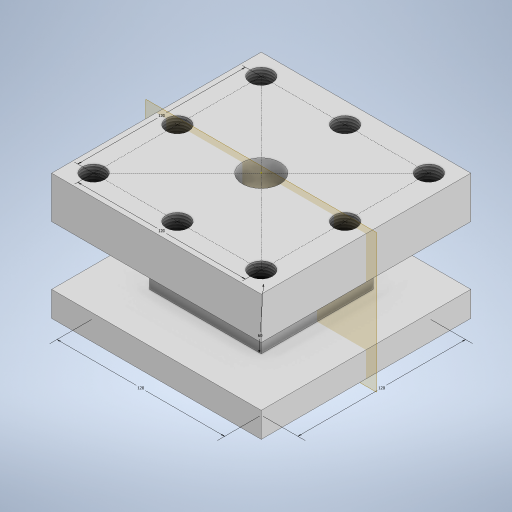
# Autodesk Inventor part: Body
Saved by Autodesk Inventor 2024 (Build 280153000, 153)
## iProperties
Created: 2023-11-09
Part Number: Body
Material: Generic
Document SubType Name: Modeling
Designer: Admin
Density: 1 g/cm^3
Appearance: Default
Author: Admin
Autodesk Inventor part; units mm, degrees
ref_plane "YZ Plane" through (0, 0, 0) normal (1, 0, 0) x (0, 1, 0)
ref_plane "XZ Plane" through (0, 0, 0) normal (0, 1, 0) x (-1, 0, 0)
sketch "Sketch1" plane through (0, 0, 0) normal (0, 1, 0) x (-1, 0, 0)
  line L0 (-75, -75) -> (75, -75)
  line L1 (75, -75) -> (75, 75)
  line L2 (75, 75) -> (-75, 75)
  line L3 (-75, 75) -> (-75, -75)
  line L4 (-75, -75) -> (75, 75) construction
  line L5 (75, -75) -> (-75, 75) construction
  point P0 (0, 0)
  dimension "d0" = 150
  dimension "d1" = 150
  constraints: 12 end point, 2 midpoint, 2 parallel, 1 horizontal, 1 perpendicular
  measures "d0" distance of L2.end L1.end
  measures "d1" distance of L1.end L0.end
extrude "Extrusion1" add sketch "Sketch1" against normal blind 18
sketch "Sketch2" plane through (0, -18, 0) normal (0, -1, 0) x (1, 0, 0)
  circle A0 centre (0, 0) radius 30
  line L0 (-60, -60) -> (60, -60) construction
  line L1 (60, -60) -> (60, 60) construction
  line L2 (60, 60) -> (-60, 60) construction
  line L3 (-60, 60) -> (-60, -60) construction
  line L4 (-60, -60) -> (60, 60) construction
  line L5 (60, -60) -> (-60, 60) construction
  dimension "d4" = 60
  dimension "d5" = 120
  dimension "d6" = 120
  constraints: 12 end point, 2 midpoint, 2 parallel, 1 centre point, 1 coincident, 1 horizontal, 1 perpendicular
  measures "d4" diameter of A0
  measures "d5" distance of L2.end L1.end
  measures "d6" distance of L1.end L0.end
extrude "Extrusion2" cut sketch "Sketch2" against normal blind 10
sketch "Sketch3" plane through (0, -18, 0) normal (0, -1, 0) x (1, 0, 0)
  line L0 (60, -60) -> (60, 60) construction
  line L1 (60, 60) -> (-60, 60) construction
  line L2 (-60, 60) -> (-60, -60) construction
  line L3 (-60, -60) -> (60, -60) construction
  point P0 (0, 0)
  point P1 (60, 0)
  point P2 (-60, 0)
  point P3 (0, 60)
  point P4 (0, -60)
  constraints: 4 midpoint
hole "Hole1" at (0, -18, 60) at (-60, -18, 0) at (0, -18, -60) at (60, -18, 0) direction (0, 1, 0) diameter 10 depth 13 tip angle 100
sketch "Sketch4" plane through (0, 0, 0) normal (0, 1, 0) x (1, 0, 0)
  line L0 (40, -40) -> (-40, -40)
  line L1 (-40, -40) -> (-40, 40)
  line L2 (-40, 40) -> (40, 40)
  line L3 (40, 40) -> (40, -40)
  line L4 (40, -40) -> (-40, 40) construction
  line L5 (-40, -40) -> (40, 40) construction
  point P0 (0, 0)
  dimension "d16" = 80
  dimension "d17" = 80
  constraints: 12 end point, 2 midpoint, 2 parallel, 1 horizontal, 1 perpendicular
  measures "d16" distance of L1.end L2.end
  measures "d17" distance of L0.end L1.end
extrude "Extrusion3" add sketch "Sketch4" along normal blind 42
sketch "Sketch5" plane through (0, 42, 0) normal (0, 1, 0) x (1, 0, 0)
  line L0 (75, -75) -> (-75, -75)
  line L1 (-75, -75) -> (-75, 75)
  line L2 (-75, 75) -> (75, 75)
  line L3 (75, 75) -> (75, -75)
  line L4 (75, -75) -> (-75, 75) construction
  line L5 (-75, -75) -> (75, 75) construction
  point P0 (0, 0)
  constraints: 12 end point, 2 midpoint, 2 parallel, 1 horizontal, 1 perpendicular
extrude "Extrusion4" add sketch "Sketch5" along normal blind 30
sketch "Sketch6" plane through (0, 72, 0) normal (0, 1, 0) x (1, 0, 0)
  circle A0 centre (0, 0) radius 13.5
  dimension "d22" = 27
  constraints: 1 centre point, 1 coincident
  measures "d22" diameter of A0
extrude "Extrusion5" cut sketch "Sketch6" against normal through all
sketch "Sketch7" plane through (0, 72, 0) normal (0, 1, 0) x (1, 0, 0)
  line L0 (60, 60) -> (-60, 60) construction
  line L1 (-60, 60) -> (-60, -60) construction
  line L2 (-60, -60) -> (60, -60) construction
  line L3 (60, -60) -> (60, 60) construction
  line L4 (60, 60) -> (-60, -60) construction
  line L5 (-60, 60) -> (60, -60) construction
  point P0 (0, 0)
  point P1 (0, 60)
  point P2 (-60, 0)
  point P3 (0, -60)
  point P4 (60, 0)
  dimension "d25" = 120
  dimension "d26" = 120
  constraints: 12 end point, 6 midpoint, 4 coincident, 2 parallel, 1 horizontal, 1 perpendicular
  measures "d25" distance of L2.end L1.end
  measures "d26" distance of L1.end L0.end
hole "Hole2" at (-60, 72, 60) at (0, 72, 60) at (60, 72, 60) at (60, 72, 0) at (60, 72, -60) at (0, 72, -60) at (-60, 72, -60) at (-60, 72, 0) direction (0, -1, 0) diameter 16 depth 30 tip angle 100
thread "Thread2" size "M16x2" class "6H" standard "ANSI Metric M Profile" length 56
thread "Thread3" size "M16x2" class "6H" standard "ANSI Metric M Profile" length 56
thread "Thread4" size "M16x2" class "6H" standard "ANSI Metric M Profile" length 56
thread "Thread5" size "M16x2" class "6H" standard "ANSI Metric M Profile" length 56
thread "Thread6" size "M16x2" class "6H" standard "ANSI Metric M Profile" length 56
thread "Thread7" size "M16x2" class "6H" standard "ANSI Metric M Profile" length 56
thread "Thread8" size "M16x2" class "6H" standard "ANSI Metric M Profile" length 56
thread "Thread9" size "M16x2" class "6H" standard "ANSI Metric M Profile" length 56
body "Solid1"
